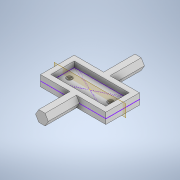
# Autodesk Inventor part: connectorToTubeBracketWithHexShaft
Saved by Autodesk Inventor 2021.1 (Build 251245010, 245A)
## iProperties
Created: 2020-07-21
Part Number: connectorToTubeBracketWithHexShaft
Material: Generic
Document SubType Name: Modeling
Designer: robst
Density: 1 g/cm^3
Appearance: Default
Author: robst
Autodesk Inventor part; units mm, degrees
ref_plane "YZ Plane" through (0, 0, 0) normal (1, 0, 0) x (0, 1, 0)
ref_plane "XZ Plane" through (0, 0, 0) normal (0, 1, 0) x (-1, 0, 0)
sketch "Sketch1" plane through (0, 0, 0) normal (0, 1, 0) x (-1, 0, 0)
  line L0 (50.8, 21.59) -> (-50.8, 21.59)
  line L1 (-50.8, 21.59) -> (-50.8, -21.59)
  line L2 (-50.8, -21.59) -> (50.8, -21.59)
  line L3 (50.8, -21.59) -> (50.8, 21.59)
  line L4 (50.8, 21.59) -> (-50.8, -21.59) construction
  line L5 (-50.8, 21.59) -> (50.8, -21.59) construction
  line L6 (60.325, 31.115) -> (-60.325, 31.115)
  line L7 (-60.325, 31.115) -> (-60.325, -31.115)
  line L8 (-60.325, -31.115) -> (60.325, -31.115)
  line L9 (60.325, -31.115) -> (60.325, 31.115)
  line L10 (60.325, 31.115) -> (-60.325, -31.115) construction
  line L11 (-60.325, 31.115) -> (60.325, -31.115) construction
  point P0 (0, 0)
  constraints: 24 end point, 4 midpoint, 4 parallel, 2 horizontal, 2 perpendicular
extrude "Extrusion1" add sketch "Sketch1" against normal blind 9.525 contours L3 L2 L1 L0 | L9 L8 L7 L6
extrude "Extrusion2" add sketch "Sketch1" along normal blind 10.16
sketch "Sketch5" plane through (0, 0, 0) normal (0, 1, 0) x (1, 0, 0)
  line L0 (-50.8, 21.59) -> (-50.8, -21.59) projected
  line L1 (50.8, -21.59) -> (50.8, 21.59) projected
  point P0 (0, 0)
  point P1 (-38.1, 0)
  point P2 (38.1, 0)
  dimension "postHoleCenter" = 12.7
  dimension "d16" = 12.7
  measures "postHoleCenter" distance from line of L0 point (-38.1, 0)
  measures "d16" distance from line of L1 point (38.1, 0)
hole "Hole1" at (-38.1, 0, 0) at (38.1, 0, 0) direction (0, -1, 0) diameter 5.1054 end through all counterbore diameter 10.16 counterbore depth 2.54 clearance for "Hex Machine Screw" size "#10" standard "Ansi Unified Screw Threads"
sketch "Sketch6" plane through (-60.325, -9.525, 31.115) normal (0, 0, 1) x (1, 0, 0)
  line L0 (0, 19.685) -> (120.65, 19.685) projected
  line L1 (66.1909, 19.685) -> (72.0568, 9.525)
  line L2 (72.0568, 9.525) -> (66.1909, -0.635)
  line L3 (66.1909, -0.635) -> (54.4591, -0.635)
  line L4 (54.4591, -0.635) -> (48.5932, 9.525)
  line L5 (48.5932, 9.525) -> (54.4591, 19.685)
  line L6 (54.4591, 19.685) -> (66.1909, 19.685)
  point P0 (60.325, 9.525)
  point P1 (60.325, 9.525)
  constraints: 12 end point, 1 coincident, 1 collinear, 13 other
extrude "Extrusion5" add sketch "Sketch6" along normal blind 57.785
mirror "Mirror2" about plane through (0, 0, 0) normal (0, 0, 1) of "Extrusion5"
equation "\"d4\" = wallThickness"
equation "\"d16\" = postHoleCenter"
equation "\"d25\" = hexExtensionLength"
equation "\"wallThickness\" = 9.525"
equation "\"outerWidth\" = innerWidth + 2 * wallThickness"
equation "\"outerLength\" = innerLength + 2 * wallThickness"
equation "\"outerHeight\" = innerDepth + wallThickness"
equation "\"shortenForTestPrint\" = 76.2"
equation "\"hexExtensionLength\" = -0.5 * outerWidth + 0.5 * maxWidth"
equation "\"maxWidth\" = 177.8"
equation "\"innerWidth\" = 43.18"
equation "\"innerLength\" = 101.6"
equation "\"innerDepth\" = 10.16"
body "Solid1"
